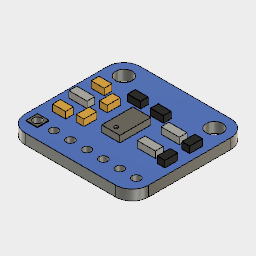
1893 Altimeter MLP3115A2 (Autodesk Fusion 360 design; units mm, degrees)
Autodesk Fusion 360 part; units mm, degrees
sketch "MPL3115A2_v0.2" plane through (0, 0, 0) normal (0, 0, 1) x (1, 0, 0)
  arc A0 (16.51, 0) -> (19.05, 2.54) centre (16.51, 2.54) ccw
  arc A1 (2.54, 17.78) -> (0, 15.24) centre (2.54, 15.24) ccw
  line L0 (19.05, 15.24) -> (19.05, 2.54)
  arc A2 (0, 2.54) -> (2.54, 0) centre (2.54, 2.54) ccw
  arc A3 (19.05, 15.24) -> (16.51, 17.78) centre (16.51, 15.24) ccw
  line L1 (2.54, 17.78) -> (16.51, 17.78)
  line L2 (0, 2.54) -> (0, 15.24)
  line L3 (16.51, 0) -> (2.54, 0)
  line L4 (1.016, 3.429) -> (1.016, 1.651)
  line L5 (1.016, 1.651) -> (2.794, 1.651)
  line L6 (2.794, 1.651) -> (2.794, 3.429)
  line L7 (1.016, 3.429) -> (1.016, 1.651)
  line L8 (1.016, 1.651) -> (2.794, 1.651)
  line L9 (2.794, 3.429) -> (1.016, 3.429)
  line L10 (2.794, 1.651) -> (2.794, 3.429)
  line L11 (2.794, 3.429) -> (1.016, 3.429)
  circle A4 centre (1.905, 2.54) radius 0.635
  circle A5 centre (4.445, 2.54) radius 0.635
  circle A6 centre (6.985, 2.54) radius 0.635
  circle A7 centre (9.525, 2.54) radius 0.635
  circle A8 centre (12.065, 2.54) radius 0.635
  circle A9 centre (14.605, 2.54) radius 0.635
  circle A10 centre (17.145, 2.54) radius 0.635
  circle A11 centre (2.54, 15.24) radius 1.27
  circle A12 centre (16.51, 15.24) radius 1.27
  dimension "d2" = 1.27
  dimension "d5" = 2.54
  dimension "d6" = 0
  dimension "d7" = 2.54
  dimension "d8" = 2.54
  measures "d2" diameter of A4
  measures "d7" diameter of A11
  measures "d8" diameter of A12
extrude "Extrude1" add sketch "MPL3115A2_v0.2" along normal blind 1.6 contours A0 A1 L0 A2 A3 L1 L2 L3 | L4 L5 L6 L7 L8 L9 L10 L11 makes body 1
extrude "Extrude2" add sketch "MPL3115A2_v0.2" along normal blind 0.1 from surface at 1.6 contours L4 L5 L6 L7 L8 L9 L10 L11 bodies 1
sketch "Sketch2" plane through (0, 0, 1.6) normal (0, 0, 1) x (-1, 0, 0)
  line L0 (-2.794, -1.651) -> (-1.016, -1.651)
  line L1 (-1.016, -1.651) -> (-1.016, -3.429)
  line L2 (-1.016, -3.429) -> (-2.794, -3.429)
  line L3 (-2.794, -3.429) -> (-2.794, -1.651)
  circle A0 centre (-17.145, -2.54) radius 0.635
  circle A1 centre (-16.51, -15.24) radius 1.27
  circle A2 centre (-9.525, -2.54) radius 0.635
  circle A3 centre (-12.065, -2.54) radius 0.635
  circle A4 centre (-2.54, -15.24) radius 1.27
  circle A5 centre (-4.445, -2.54) radius 0.635
  circle A6 centre (-14.605, -2.54) radius 0.635
  circle A7 centre (-6.985, -2.54) radius 0.635
  arc A8 (-19.05, -15.24) -> (-16.51, -17.78) centre (-16.51, -15.24) ccw
  line L4 (-16.51, -17.78) -> (-2.54, -17.78)
  arc A9 (-2.54, -17.78) -> (0, -15.24) centre (-2.54, -15.24) ccw
  line L5 (0, -15.24) -> (0, -2.54)
  arc A10 (0, -2.54) -> (-2.54, 0) centre (-2.54, -2.54) ccw
  line L6 (-2.54, 0) -> (-16.51, 0)
  arc A11 (-16.51, 0) -> (-19.05, -2.54) centre (-16.51, -2.54) ccw
  line L7 (-19.05, -2.54) -> (-19.05, -15.24)
  line L8 (-11.179, -5.982) -> (-8.379, -5.982)
  line L9 (-8.379, -5.982) -> (-8.379, -10.782)
  line L10 (-8.379, -10.782) -> (-11.179, -10.782)
  line L11 (-11.179, -10.782) -> (-11.179, -5.982)
  line L12 (-11.179, -5.982) -> (-8.379, -10.782) construction
  line L13 (-8.379, -5.982) -> (-11.179, -10.782) construction
  line L14 (-4.067, -8.036) -> (-1.267, -8.036)
  line L15 (-1.267, -8.036) -> (-1.267, -9.236)
  line L16 (-1.267, -9.236) -> (-4.067, -9.236)
  line L17 (-4.067, -9.236) -> (-4.067, -8.036)
  line L18 (-4.067, -8.036) -> (-1.267, -9.236) construction
  line L19 (-1.267, -8.036) -> (-4.067, -9.236) construction
  line L20 (-1.794, -4.988) -> (-3.794, -4.988)
  line L21 (-3.794, -4.988) -> (-3.794, -6.188)
  line L22 (-3.794, -6.188) -> (-1.794, -6.188)
  line L23 (-1.794, -6.188) -> (-1.794, -4.988)
  line L24 (-1.794, -4.988) -> (-3.794, -6.188) construction
  line L25 (-3.794, -4.988) -> (-1.794, -6.188) construction
  line L26 (-3.667, -11.076) -> (-1.667, -11.076)
  line L27 (-1.667, -11.076) -> (-1.667, -12.276)
  line L28 (-1.667, -12.276) -> (-3.667, -12.276)
  line L29 (-3.667, -12.276) -> (-3.667, -11.076)
  line L30 (-3.667, -11.076) -> (-1.667, -12.276) construction
  line L31 (-1.667, -11.076) -> (-3.667, -12.276) construction
  line L32 (-8.239, -12.1) -> (-6.239, -12.1)
  line L33 (-6.239, -12.1) -> (-6.239, -13.3)
  line L34 (-6.239, -13.3) -> (-8.239, -13.3)
  line L35 (-8.239, -13.3) -> (-8.239, -12.1)
  line L36 (-8.239, -12.1) -> (-6.239, -13.3) construction
  line L37 (-6.239, -12.1) -> (-8.239, -13.3) construction
  line L38 (-11.922, -11.973) -> (-9.922, -11.973)
  line L39 (-9.922, -11.973) -> (-9.922, -13.173)
  line L40 (-9.922, -13.173) -> (-11.922, -13.173)
  line L41 (-11.922, -13.173) -> (-11.922, -11.973)
  line L42 (-11.922, -11.973) -> (-9.922, -13.173) construction
  line L43 (-9.922, -11.973) -> (-11.922, -13.173) construction
  line L44 (-16.005, -10.322) -> (-13.205, -10.322)
  line L45 (-13.205, -10.322) -> (-13.205, -11.522)
  line L46 (-13.205, -11.522) -> (-16.005, -11.522)
  line L47 (-16.005, -11.522) -> (-16.005, -10.322)
  line L48 (-16.005, -10.322) -> (-13.205, -11.522) construction
  line L49 (-13.205, -10.322) -> (-16.005, -11.522) construction
  line L50 (-16.005, -6.639) -> (-13.205, -6.639)
  line L51 (-13.205, -6.639) -> (-13.205, -7.839)
  line L52 (-13.205, -7.839) -> (-16.005, -7.839)
  line L53 (-16.005, -7.839) -> (-16.005, -6.639)
  line L54 (-16.005, -6.639) -> (-13.205, -7.839) construction
  line L55 (-13.205, -6.639) -> (-16.005, -7.839) construction
  line L56 (-16.799, -9.922) -> (-17.999, -9.922)
  line L57 (-17.999, -9.922) -> (-17.999, -11.922)
  line L58 (-17.999, -11.922) -> (-16.799, -11.922)
  line L59 (-16.799, -11.922) -> (-16.799, -9.922)
  line L60 (-16.799, -9.922) -> (-17.999, -11.922) construction
  line L61 (-17.999, -9.922) -> (-16.799, -11.922) construction
  line L62 (-16.799, -6.112) -> (-17.999, -6.112)
  line L63 (-17.999, -6.112) -> (-17.999, -8.112)
  line L64 (-17.999, -8.112) -> (-16.799, -8.112)
  line L65 (-16.799, -8.112) -> (-16.799, -6.112)
  line L66 (-16.799, -6.112) -> (-17.999, -8.112) construction
  line L67 (-17.999, -6.112) -> (-16.799, -8.112) construction
  line L68 (-4.988, -9.033) -> (-6.188, -9.033)
  line L69 (-6.188, -9.033) -> (-6.188, -11.033)
  line L70 (-6.188, -11.033) -> (-4.988, -11.033)
  line L71 (-4.988, -11.033) -> (-4.988, -9.033)
  line L72 (-4.988, -9.033) -> (-6.188, -11.033) construction
  line L73 (-6.188, -9.033) -> (-4.988, -11.033) construction
  line L74 (-5.023, -5.396) -> (-6.223, -5.396)
  line L75 (-6.223, -5.396) -> (-6.223, -7.396)
  line L76 (-6.223, -7.396) -> (-5.023, -7.396)
  line L77 (-5.023, -7.396) -> (-5.023, -5.396)
  line L78 (-5.023, -5.396) -> (-6.223, -7.396) construction
  line L79 (-6.223, -5.396) -> (-5.023, -7.396) construction
  point P0 (-9.779, -8.382)
  point P1 (-2.667, -8.636)
  point P2 (-2.794, -5.588)
  point P3 (-2.667, -11.676)
  point P4 (-7.239, -12.7)
  point P5 (-10.922, -12.573)
  point P6 (-14.605, -10.922)
  point P7 (-14.605, -7.239)
  point P8 (-17.399, -10.922)
  point P9 (-17.399, -7.112)
  point P10 (-5.588, -10.033)
  point P11 (-5.623, -6.396)
  dimension "d19" = 4.8
  dimension "d20" = 2.8
  dimension "d21" = 8.382
  dimension "d22" = 9.779
  dimension "d23" = 2.8
  dimension "d24" = 1.2
  dimension "d25" = 2.667
  dimension "d26" = 8.636
  dimension "d27" = 2
  dimension "d28" = 1.2
  dimension "d29" = 2.794
  dimension "d30" = 5.588
  dimension "d31" = 2
  dimension "d32" = 1.2
  dimension "d33" = 2.667
  dimension "d34" = 11.676
  dimension "d35" = 2
  dimension "d36" = 1.2
  dimension "d37" = 12.7
  dimension "d38" = 7.239
  dimension "d39" = 1.2
  dimension "d40" = 2
  dimension "d41" = 12.573
  dimension "d42" = 10.922
  dimension "d43" = 2.8
  dimension "d44" = 1.2
  dimension "d45" = 2.8
  dimension "d46" = 1.2
  dimension "d47" = 2
  dimension "d48" = 1.2
  dimension "d49" = 2
  dimension "d50" = 1.2
  dimension "d51" = 10.922
  dimension "d52" = 14.605
  dimension "d53" = 7.239
  dimension "d54" = 14.605
  dimension "d55" = 10.922
  dimension "d56" = 17.399
  dimension "d57" = 7.112
  dimension "d58" = 17.399
  dimension "d66" = 2
  dimension "d67" = 1.2
  dimension "d68" = 2
  dimension "d69" = 1.2
  dimension "d70" = 5.588
  dimension "d71" = 10.033
  dimension "d72" = 5.623
  dimension "d73" = 6.396
  measures "d19" distance of L8.end L9.end
  measures "d20" distance of L9.end L10.end
  measures "d21" distance of L6 P0
  measures "d22" distance of L5 P0
  measures "d23" distance of L15.end L16.end
  measures "d24" distance of L14.end L15.end
  measures "d25" distance of L5 P1
  measures "d26" distance of L6 P1
  measures "d27" distance of L21.end L22.end
  measures "d28" distance of L20.end L21.end
  measures "d29" distance of L5 P2
  measures "d30" distance of L6 P2
  measures "d31" distance of L27.end L28.end
  measures "d32" distance of L26.end L27.end
  measures "d33" distance of L5 P3
  measures "d34" distance of L6 P3
  measures "d35" distance of L33.end L34.end
  measures "d36" distance of L32.end L33.end
  measures "d37" distance of L6 P4
  measures "d38" distance of L5 P4
  measures "d39" distance of L38.end L39.end
  measures "d40" distance of L39.end L40.end
  measures "d41" distance of L6 P5
  measures "d42" distance of L5 P5
  measures "d43" distance of L45.end L46.end
  measures "d44" distance of L44.end L45.end
  measures "d45" distance of L51.end L52.end
  measures "d46" distance of L50.end L51.end
  measures "d47" distance of L56.end L57.end
  measures "d48" distance of L57.end L58.end
  measures "d49" distance of L62.end L63.end
  measures "d50" distance of L63.end L64.end
  measures "d51" distance of L6 P6
  measures "d52" distance of L5 P6
  measures "d53" distance of L6 P7
  measures "d54" distance of L5 P7
  measures "d55" distance of L6 P8
  measures "d56" distance of L5 P8
  measures "d57" distance of L6 P9
  measures "d58" distance of L5 P9
  measures "d66" distance of L68.end L69.end
  measures "d67" distance of L69.end L70.end
  measures "d68" distance of L74.end L75.end
  measures "d69" distance of L75.end L76.end
  measures "d70" distance of L5 P10
  measures "d71" distance of L6 P10
  measures "d72" distance of L5 P11
  measures "d73" distance of L6 P11
extrude "Extrude3" add sketch "Sketch2" along normal blind 1 separate body contours L8 L9 L10 L11 | L14 L15 L16 L17 | L20 L21 L22 L23 | L26 L27 L28 L29 | L32 L33 L34 L35 | L38 L39 L40 L41 | L44 L45 L46 L47 | L50 L51 L52 L53 | L56 L57 L58 L59 | L62 L63 L64 L65 | L68 L69 L70 L71 | L74 L75 L76 L77 makes body 2 at (17.199, 7.4453, 1.6) makes body 3 at (11.2553, 12.773, 1.6) makes body 4 at (3.1273, 5.388, 1.6) makes body 5 at (3.1337, 8.436, 1.6) makes body 6 at (15.0717, 10.722, 1.6) makes body 7 at (5.823, 6.0627, 1.6) makes body 8 at (15.0717, 7.039, 1.6) makes body 9 at (7.5723, 12.5, 1.6) makes body 10 at (10.2457, 7.582, 1.6) makes body 11 at (3.0003, 11.876, 1.6) makes body 12 at (17.199, 11.2553, 1.6) makes body 13 at (5.788, 9.6997, 1.6)
sketch "Sketch3" plane through (0, 0, 2.6) normal (0, 0, 1) x (-1, 0, 0)
  line L0 (-11.179, -10.782) -> (-8.379, -10.782)
  line L1 (-8.379, -10.782) -> (-8.379, -5.982)
  line L2 (-8.379, -5.982) -> (-11.179, -5.982)
  line L3 (-11.179, -5.982) -> (-11.179, -10.782)
  circle A0 centre (-9.779, -6.782) radius 0.3
  dimension "d61" = 0.6
  dimension "d65" = 0.8
  measures "d61" diameter of A0
  measures "d65" distance of L2 A0.centre
extrude "Extrude4" cut sketch "Sketch3" against normal blind 0.2 contours A0 bodies 8 4 1 6 2 12 11 5 3 9 10
